Autodesk Inventor part; units mm, degrees
(part 2 of 2)
sketch "Sketch3" plane through (0, 0, -3.4) normal (0, 0, -1) x (-1, 0, 0)
  line L0 (0, 0.65) -> (23.75, 0.65)
  line L1 (23.75, 0.65) -> (23.75, 66.4871)
  line L2 (23.75, 66.4871) -> (0, 66.4871)
  line L3 (0, 66.4871) -> (0, 0.65)
  circle A0 centre (13, 35.9222) radius 9.6 construction
  circle A1 centre (9.652, 48.0693) radius 8 construction
  circle A2 centre (9.652, 48.0693) radius 8.4
  circle A3 centre (13, 35.9222) radius 10
  circle A4 centre (15.35, 56.2871) radius 5 projected
  circle A5 centre (9.652, 48.0693) radius 1.25 construction
  arc A6 (10.4245, 56.0319) -> (9.9568, 54.9375) centre (14.7581, 53.5328) ccw construction
  arc A7 (9.9568, 54.9375) -> (9.5969, 54.944) centre (9.652, 48.0693) ccw construction
  arc A8 (9.5969, 54.944) -> (9.1694, 56.0547) centre (4.7478, 53.7148) ccw construction
  arc A9 (9.1694, 56.0547) -> (8.7521, 56.0185) centre (9.652, 48.0693) ccw construction
  arc A10 (8.7521, 56.0185) -> (8.5222, 54.8508) centre (13.5106, 54.4751) ccw construction
  arc A11 (8.5222, 54.8508) -> (8.1688, 54.7824) centre (9.652, 48.0693) ccw construction
  arc A12 (8.1688, 54.7824) -> (7.5196, 55.7798) centre (3.6812, 52.5718) ccw construction
  arc A13 (7.5196, 55.7798) -> (7.119, 55.6577) centre (9.652, 48.0693) ccw construction
  arc A14 (7.119, 55.6577) -> (7.1369, 54.4677) centre (12.0944, 55.1373) ccw construction
  arc A15 (7.1369, 54.4677) -> (6.8055, 54.3273) centre (9.652, 48.0693) ccw construction
  arc A16 (6.8055, 54.3273) -> (5.9631, 55.168) centre (2.8755, 51.232) ccw construction
  arc A17 (5.9631, 55.168) -> (5.5966, 54.9652) centre (9.652, 48.0693) ccw construction
  arc A18 (5.5966, 54.9652) -> (5.8615, 53.805) centre (10.5715, 55.4907) ccw construction
  arc A19 (5.8615, 53.805) -> (5.5666, 53.5987) centre (9.652, 48.0693) ccw construction
  arc A20 (5.5666, 53.5987) -> (4.5678, 54.2459) centre (2.366, 49.754) ccw construction
  arc A21 (4.5678, 54.2459) -> (4.2515, 53.9714) centre (9.652, 48.0693) ccw construction
  arc A22 (4.2515, 53.9714) -> (4.7519, 52.8916) centre (9.0084, 55.5197) ccw construction
  arc A23 (4.7519, 52.8916) -> (4.5062, 52.6285) centre (9.652, 48.0693) ccw construction
  arc A24 (4.5062, 52.6285) -> (3.3947, 53.0539) centre (2.175, 48.2023) ccw construction
  arc A25 (3.3947, 53.0539) -> (3.1424, 52.7196) centre (9.652, 48.0693) ccw construction
  arc A26 (3.1424, 52.7196) -> (3.8563, 51.7674) centre (7.4735, 55.2231) ccw construction
  arc A27 (3.8563, 51.7674) -> (3.6707, 51.459) centre (9.652, 48.0693) ccw construction
  arc A28 (3.6707, 51.459) -> (2.4951, 51.644) centre (2.3107, 46.6449) ccw construction
  arc A29 (2.4951, 51.644) -> (2.3178, 51.2646) centre (9.652, 48.0693) ccw construction
  arc A30 (2.3178, 51.2646) -> (3.2141, 50.4816) centre (6.0337, 54.6138) ccw construction
  arc A31 (3.2141, 50.4816) -> (3.0967, 50.1413) centre (9.652, 48.0693) ccw construction
  arc A32 (3.0967, 50.1413) -> (1.9082, 50.0779) centre (2.7673, 45.1497) ccw construction
  arc A33 (1.9082, 50.0779) -> (1.8137, 49.6699) centre (9.652, 48.0693) ccw construction
  arc A34 (1.8137, 49.6699) -> (2.8532, 49.0904) centre (4.7521, 53.7185) ccw construction
  arc A35 (2.8532, 49.0904) -> (2.8091, 48.7331) centre (9.652, 48.0693) ccw construction
  arc A36 (2.8091, 48.7331) -> (1.6598, 48.424) centre (3.5247, 43.7821) ccw construction
  arc A37 (1.6598, 48.424) -> (1.6522, 48.0052) centre (9.652, 48.0693) ccw construction
  arc A38 (1.6522, 48.0052) -> (2.7895, 47.6545) centre (3.6846, 52.5763) ccw construction
  arc A39 (2.7895, 47.6545) -> (2.8206, 47.2959) centre (9.652, 48.0693) ccw construction
  arc A40 (2.8206, 47.2959) -> (1.7607, 46.7546) centre (4.55, 42.6018) ccw construction
  arc A41 (1.7607, 46.7546) -> (1.8404, 46.3434) centre (9.652, 48.0693) ccw construction
  arc A42 (1.8404, 46.3434) -> (3.0257, 46.2368) centre (2.8779, 51.2371) ccw construction
  arc A43 (3.0257, 46.2368) -> (3.1307, 45.8925) centre (9.652, 48.0693) ccw construction
  arc A44 (3.1307, 45.8925) -> (2.2065, 45.1426) centre (5.7982, 41.6605) ccw construction
  arc A45 (2.2065, 45.1426) -> (2.3699, 44.757) centre (9.652, 48.0693) ccw construction
  arc A46 (2.3699, 44.757) -> (3.5515, 44.8991) centre (2.3673, 49.7595) ccw construction
  arc A47 (3.5515, 44.8991) -> (3.7258, 44.5842) centre (9.652, 48.0693) ccw construction
  arc A48 (3.7258, 44.5842) -> (2.9777, 43.6586) centre (7.2149, 40.9993) ccw construction
  arc A49 (2.9777, 43.6586) -> (3.2177, 43.3153) centre (9.652, 48.0693) ccw construction
  arc A50 (3.2177, 43.3153) -> (4.3439, 43.7001) centre (2.1751, 48.208) ccw construction
  arc A51 (4.3439, 43.7001) -> (4.5798, 43.4282) centre (9.652, 48.0693) ccw construction
  arc A52 (4.5798, 43.4282) -> (4.0406, 42.3673) centre (8.7381, 40.6471) ccw construction
  arc A53 (4.0406, 42.3673) -> (4.3467, 42.0814) centre (9.652, 48.0693) ccw construction
  arc A54 (4.3467, 42.0814) -> (5.3683, 42.6919) centre (2.3096, 46.6504) ccw construction
  arc A55 (5.3683, 42.6919) -> (5.6556, 42.4751) centre (9.652, 48.0693) ccw construction
  arc A56 (5.6556, 42.4751) -> (5.3487, 41.3252) centre (10.3012, 40.6193) ccw construction
  arc A57 (5.3487, 41.3252) -> (5.7076, 41.1093) centre (9.652, 48.0693) ccw construction
  arc A58 (5.7076, 41.1093) -> (6.5799, 41.9188) centre (2.7651, 45.1549) ccw construction
  arc A59 (6.5799, 41.9188) -> (6.906, 41.7665) centre (9.652, 48.0693) ccw construction
  arc A60 (6.906, 41.7665) -> (6.8449, 40.5779) centre (11.8359, 40.9171) ccw construction
  arc A61 (6.8449, 40.5779) -> (7.2408, 40.4413) centre (9.652, 48.0693) ccw construction
  arc A62 (7.2408, 40.4413) -> (7.9258, 41.4145) centre (3.5215, 43.7867) ccw construction
  arc A63 (7.9258, 41.4145) -> (8.2764, 41.3333) centre (9.652, 48.0693) ccw construction
  arc A64 (8.2764, 41.3333) -> (8.4638, 40.158) centre (13.2752, 41.5275) ccw construction
  arc A65 (8.4638, 40.158) -> (8.8795, 40.1066) centre (9.652, 48.0693) ccw construction
  arc A66 (8.8795, 40.1066) -> (9.3471, 41.201) centre (4.5458, 42.6057) ccw construction
  arc A67 (9.3471, 41.201) -> (9.707, 41.1945) centre (9.652, 48.0693) ccw construction
  arc A68 (9.707, 41.1945) -> (10.1346, 40.0838) centre (14.5562, 42.4237) ccw construction
  arc A69 (10.1346, 40.0838) -> (10.5519, 40.12) centre (9.652, 48.0693) ccw construction
  arc A70 (10.5519, 40.12) -> (10.7818, 41.2877) centre (5.7934, 41.6635) ccw construction
  arc A71 (10.7818, 41.2877) -> (11.1351, 41.3561) centre (9.652, 48.0693) ccw construction
  arc A72 (11.1351, 41.3561) -> (11.7843, 40.3587) centre (15.6228, 43.5667) ccw construction
  arc A73 (11.7843, 40.3587) -> (12.1849, 40.4808) centre (9.652, 48.0693) ccw construction
  arc A74 (12.1849, 40.4808) -> (12.167, 41.6708) centre (7.2095, 41.0012) ccw construction
  arc A75 (12.167, 41.6708) -> (12.4985, 41.8112) centre (9.652, 48.0693) ccw construction
  arc A76 (12.4985, 41.8112) -> (13.3408, 40.9705) centre (16.4284, 44.9065) ccw construction
  arc A77 (13.3408, 40.9705) -> (13.7073, 41.1733) centre (9.652, 48.0693) ccw construction
  arc A78 (13.7073, 41.1733) -> (13.4424, 42.3336) centre (8.7324, 40.6478) ccw construction
  arc A79 (13.4424, 42.3336) -> (13.7374, 42.5398) centre (9.652, 48.0693) ccw construction
  arc A80 (13.7374, 42.5398) -> (14.7361, 41.8926) centre (16.9379, 46.3845) ccw construction
  arc A81 (14.7361, 41.8926) -> (15.0524, 42.1671) centre (9.652, 48.0693) ccw construction
  arc A82 (15.0524, 42.1671) -> (14.5521, 43.247) centre (10.2955, 40.6188) ccw construction
  arc A83 (14.5521, 43.247) -> (14.7977, 43.51) centre (9.652, 48.0693) ccw construction
  arc A84 (14.7977, 43.51) -> (15.9092, 43.0846) centre (17.129, 47.9362) ccw construction
  arc A85 (15.9092, 43.0846) -> (16.1615, 43.4189) centre (9.652, 48.0693) ccw construction
  arc A86 (16.1615, 43.4189) -> (15.4476, 44.3711) centre (11.8305, 40.9154) ccw construction
  arc A87 (15.4476, 44.3711) -> (15.6332, 44.6795) centre (9.652, 48.0693) ccw construction
  arc A88 (15.6332, 44.6795) -> (16.8089, 44.4945) centre (16.9932, 49.4936) ccw construction
  arc A89 (16.8089, 44.4945) -> (16.9861, 44.874) centre (9.652, 48.0693) ccw construction
  arc A90 (16.9861, 44.874) -> (16.0899, 45.6569) centre (13.2702, 41.5247) ccw construction
  arc A91 (16.0899, 45.6569) -> (16.2073, 45.9972) centre (9.652, 48.0693) ccw construction
  arc A92 (16.2073, 45.9972) -> (17.3957, 46.0606) centre (16.5367, 50.9889) ccw construction
  arc A93 (17.3957, 46.0606) -> (17.4902, 46.4687) centre (9.652, 48.0693) ccw construction
  arc A94 (17.4902, 46.4687) -> (16.4507, 47.0482) centre (14.5519, 42.42) ccw construction
  arc A95 (16.4507, 47.0482) -> (16.4948, 47.4054) centre (9.652, 48.0693) ccw construction
  arc A96 (16.4948, 47.4054) -> (17.6441, 47.7145) centre (15.7792, 52.3565) ccw construction
  arc A97 (17.6441, 47.7145) -> (17.6517, 48.1333) centre (9.652, 48.0693) ccw construction
  arc A98 (17.6517, 48.1333) -> (16.5144, 48.484) centre (15.6193, 43.5622) ccw construction
  arc A99 (16.5144, 48.484) -> (16.4833, 48.8426) centre (9.652, 48.0693) ccw construction
  arc A100 (16.4833, 48.8426) -> (17.5432, 49.3839) centre (14.7539, 53.5367) ccw construction
  arc A101 (17.5432, 49.3839) -> (17.4636, 49.7951) centre (9.652, 48.0693) ccw construction
  arc A102 (17.4636, 49.7951) -> (16.2783, 49.9017) centre (16.426, 44.9014) ccw construction
  arc A103 (16.2783, 49.9017) -> (16.1733, 50.246) centre (9.652, 48.0693) ccw construction
  arc A104 (16.1733, 50.246) -> (17.0974, 50.9959) centre (13.5057, 54.478) ccw construction
  arc A105 (17.0974, 50.9959) -> (16.9341, 51.3815) centre (9.652, 48.0693) ccw construction
  arc A106 (16.9341, 51.3815) -> (15.7525, 51.2394) centre (16.9366, 46.379) ccw construction
  arc A107 (15.7525, 51.2394) -> (15.5782, 51.5543) centre (9.652, 48.0693) ccw construction
  arc A108 (15.5782, 51.5543) -> (16.3262, 52.4799) centre (12.089, 55.1392) ccw construction
  arc A109 (16.3262, 52.4799) -> (16.0863, 52.8232) centre (9.652, 48.0693) ccw construction
  arc A110 (16.0863, 52.8232) -> (14.96, 52.4385) centre (17.1289, 47.9305) ccw construction
  arc A111 (14.96, 52.4385) -> (14.7241, 52.7103) centre (9.652, 48.0693) ccw construction
  arc A112 (14.7241, 52.7103) -> (15.2634, 53.7712) centre (10.5659, 55.4914) ccw construction
  arc A113 (15.2634, 53.7712) -> (14.9573, 54.0571) centre (9.652, 48.0693) ccw construction
  arc A114 (14.9573, 54.0571) -> (13.9356, 53.4466) centre (16.9943, 49.4881) ccw construction
  arc A115 (13.9356, 53.4466) -> (13.6483, 53.6634) centre (9.652, 48.0693) ccw construction
  arc A116 (13.6483, 53.6634) -> (13.9552, 54.8133) centre (9.0028, 55.5192) ccw construction
  arc A117 (13.9552, 54.8133) -> (13.5964, 55.0293) centre (9.652, 48.0693) ccw construction
  arc A118 (13.5964, 55.0293) -> (12.724, 54.2197) centre (16.5389, 50.9836) ccw construction
  arc A119 (12.724, 54.2197) -> (12.3979, 54.3721) centre (9.652, 48.0693) ccw construction
  arc A120 (12.3979, 54.3721) -> (12.459, 55.5606) centre (7.468, 55.2214) ccw construction
  arc A121 (12.459, 55.5606) -> (12.0631, 55.6973) centre (9.652, 48.0693) ccw construction
  arc A122 (12.0631, 55.6973) -> (11.3781, 54.724) centre (15.7825, 52.3518) ccw construction
  arc A123 (11.3781, 54.724) -> (11.0275, 54.8052) centre (9.652, 48.0693) ccw construction
  arc A124 (11.0275, 54.8052) -> (10.8402, 55.9805) centre (6.0287, 54.6111) ccw construction
  arc A125 (10.8402, 55.9805) -> (10.4245, 56.0319) centre (9.652, 48.0693) ccw construction
  arc A126 (10.4239, 28.0847) -> (10.4838, 26.6578) centre (16.409, 27.6212) ccw construction
  arc A127 (10.4838, 26.6578) -> (10.9721, 26.5388) centre (13, 35.9222) ccw construction
  arc A128 (10.9721, 26.5388) -> (11.6817, 27.7782) centre (6.1543, 30.12) ccw construction
  arc A129 (11.6817, 27.7782) -> (12.1097, 27.7204) centre (13, 35.9222) ccw construction
  arc A130 (12.1097, 27.7204) -> (12.465, 26.3371) centre (18.0604, 28.5113) ccw construction
  arc A131 (12.465, 26.3371) -> (12.9673, 26.3223) centre (13, 35.9222) ccw construction
  arc A132 (12.9673, 26.3223) -> (13.4037, 27.6821) centre (7.5102, 28.8235) ccw construction
  arc A133 (13.4037, 27.6821) -> (13.8344, 27.7145) centre (13, 35.9222) ccw construction
  arc A134 (13.8344, 27.7145) -> (14.4695, 26.4353) centre (19.4907, 29.7254) ccw construction
  arc A135 (14.4695, 26.4353) -> (14.964, 26.5253) centre (13, 35.9222) ccw construction
  arc A136 (14.964, 26.5253) -> (15.1081, 27.9461) centre (9.1061, 27.8373) ccw construction
  arc A137 (15.1081, 27.9461) -> (15.5227, 28.0674) centre (13, 35.9222) ccw construction
  arc A138 (15.5227, 28.0674) -> (16.4098, 26.9482) centre (20.6372, 31.2103) ccw construction
  arc A139 (16.4098, 26.9482) -> (16.8748, 27.1389) centre (13, 35.9222) ccw construction
  arc A140 (16.8748, 27.1389) -> (16.7204, 28.5587) centre (10.8721, 27.2043) ccw construction
  arc A141 (16.7204, 28.5587) -> (17.1007, 28.7635) centre (13, 35.9222) ccw construction
  arc A142 (17.1007, 28.7635) -> (18.2011, 27.8532) centre (21.45, 32.9011) ccw construction
  arc A143 (18.2011, 27.8532) -> (18.6163, 28.1365) centre (13, 35.9222) ccw construction
  arc A144 (18.6163, 28.1365) -> (18.17, 29.4931) centre (12.7312, 26.9524) ccw construction
  arc A145 (18.17, 29.4931) -> (18.4994, 29.7725) centre (13, 35.9222) ccw construction
  arc A146 (18.4994, 29.7725) -> (19.7651, 29.1109) centre (21.8934, 34.724) ccw construction
  arc A147 (19.7651, 29.1109) -> (20.1123, 29.4743) centre (13, 35.9222) ccw construction
  arc A148 (20.1123, 29.4743) -> (19.3937, 30.7085) centre (14.602, 27.0926) ccw construction
  arc A149 (19.3937, 30.7085) -> (19.6578, 31.0503) centre (13, 35.9222) ccw construction
  arc A150 (19.6578, 31.0503) -> (21.0334, 30.6663) centre (21.9482, 36.5992) ccw construction
  arc A151 (21.0334, 30.6663) -> (21.2975, 31.0939) centre (13, 35.9222) ccw construction
  arc A152 (21.2975, 31.0939) -> (20.338, 32.1518) centre (16.4027, 27.6186) ccw construction
  arc A153 (20.338, 32.1518) -> (20.5253, 32.541) centre (13, 35.9222) ccw construction
  arc A154 (20.5253, 32.541) -> (21.9506, 32.4514) centre (21.6119, 38.4449) ccw construction
  arc A155 (21.9506, 32.4514) -> (22.12, 32.9246) centre (13, 35.9222) ccw construction
  arc A156 (22.12, 32.9246) -> (20.9616, 33.7599) centre (18.0548, 28.5075) ccw construction
  arc A157 (20.9616, 33.7599) -> (21.0638, 34.1795) centre (13, 35.9222) ccw construction
  arc A158 (21.0638, 34.1795) -> (22.4766, 34.3882) centre (20.8992, 40.1803) ccw construction
  arc A159 (22.4766, 34.3882) -> (22.5439, 34.8863) centre (13, 35.9222) ccw construction
  arc A160 (22.5439, 34.8863) -> (21.2372, 35.4624) centre (19.486, 29.7205) ccw construction
  arc A161 (21.2372, 35.4624) -> (21.25, 35.8941) centre (13, 35.9222) ccw construction
  arc A162 (21.25, 35.8941) -> (22.5885, 36.392) centre (19.8413, 41.7296) ccw construction
  arc A163 (22.5885, 36.392) -> (22.5508, 36.8932) centre (13, 35.9222) ccw construction
  arc A164 (22.5508, 36.8932) -> (21.1528, 37.1851) centre (20.6336, 31.2045) ccw construction
  arc A165 (21.1528, 37.1851) -> (21.0755, 37.61) centre (13, 35.9222) ccw construction
  arc A166 (21.0755, 37.61) -> (22.2813, 38.3753) centre (18.4844, 43.0251) ccw construction
  arc A167 (22.2813, 38.3753) -> (22.1402, 38.8577) centre (13, 35.9222) ccw construction
  arc A168 (22.1402, 38.8577) -> (20.7121, 38.8525) centre (21.4477, 32.8947) ccw construction
  arc A169 (20.7121, 38.8525) -> (20.5481, 39.2521) centre (13, 35.9222) ccw construction
  arc A170 (20.5481, 39.2521) -> (21.5684, 40.2514) centre (16.8878, 44.0101) ccw construction
  arc A171 (21.5684, 40.2514) -> (21.3301, 40.6939) centre (13, 35.9222) ccw construction
  arc A172 (21.3301, 40.6939) -> (19.9343, 40.3919) centre (21.8925, 34.7172) ccw construction
  arc A173 (19.9343, 40.3919) -> (19.6909, 40.7487) centre (13, 35.9222) ccw construction
  arc A174 (19.6909, 40.7487) -> (20.4811, 41.9383) centre (15.1213, 44.6417) ccw construction
  arc A175 (20.4811, 41.9383) -> (20.156, 42.3216) centre (13, 35.9222) ccw construction
  arc A176 (20.156, 42.3216) -> (18.8534, 41.736) centre (21.9487, 36.5924) ccw construction
  arc A177 (18.8534, 41.736) -> (18.5412, 42.0343) centre (13, 35.9222) ccw construction
  arc A178 (18.5412, 42.0343) -> (19.0668, 43.3622) centre (13.262, 44.8922) ccw construction
  arc A179 (19.0668, 43.3622) -> (18.6691, 43.6695) centre (13, 35.9222) ccw construction
  arc A180 (18.6691, 43.6695) -> (17.5168, 42.8259) centre (21.6138, 38.4383) ccw construction
  arc A181 (17.5168, 42.8259) -> (17.1493, 43.0528) centre (13, 35.9222) ccw construction
  arc A182 (17.1493, 43.0528) -> (17.3874, 44.461) centre (11.3913, 44.7507) ccw construction
  arc A183 (17.3874, 44.461) -> (16.9345, 44.6789) centre (13, 35.9222) ccw construction
  arc A184 (16.9345, 44.6789) -> (15.9827, 43.6141) centre (20.9025, 40.1743) ccw construction
  arc A185 (15.9827, 43.6141) -> (15.5761, 43.7597) centre (13, 35.9222) ccw construction
  arc A186 (15.5761, 43.7597) -> (15.5162, 45.1866) centre (9.591, 44.2233) ccw construction
  arc A187 (15.5162, 45.1866) -> (15.0279, 45.3056) centre (13, 35.9222) ccw construction
  arc A188 (15.0279, 45.3056) -> (14.3183, 44.0662) centre (19.8457, 41.7244) ccw construction
  arc A189 (14.3183, 44.0662) -> (13.8903, 44.124) centre (13, 35.9222) ccw construction
  arc A190 (13.8903, 44.124) -> (13.535, 45.5073) centre (7.9396, 43.3331) ccw construction
  arc A191 (13.535, 45.5073) -> (13.0327, 45.5222) centre (13, 35.9222) ccw construction
  arc A192 (13.0327, 45.5222) -> (12.5963, 44.1623) centre (18.4898, 43.0209) ccw construction
  arc A193 (12.5963, 44.1623) -> (12.1656, 44.1299) centre (13, 35.9222) ccw construction
  arc A194 (12.1656, 44.1299) -> (11.5305, 45.4091) centre (6.5093, 42.119) ccw construction
  arc A195 (11.5305, 45.4091) -> (11.036, 45.3192) centre (13, 35.9222) ccw construction
  arc A196 (11.036, 45.3192) -> (10.8919, 43.8983) centre (16.8939, 44.0072) ccw construction
  arc A197 (10.8919, 43.8983) -> (10.4773, 43.7771) centre (13, 35.9222) ccw construction
  arc A198 (10.4773, 43.7771) -> (9.5902, 44.8962) centre (5.3628, 40.6341) ccw construction
  arc A199 (9.5902, 44.8962) -> (9.1252, 44.7055) centre (13, 35.9222) ccw construction
  arc A200 (9.1252, 44.7055) -> (9.2796, 43.2857) centre (15.1279, 44.6401) ccw construction
  arc A201 (9.2796, 43.2857) -> (8.8993, 43.0809) centre (13, 35.9222) ccw construction
  arc A202 (8.8993, 43.0809) -> (7.7989, 43.9912) centre (4.55, 38.9433) ccw construction
  arc A203 (7.7989, 43.9912) -> (7.3837, 43.7079) centre (13, 35.9222) ccw construction
  arc A204 (7.3837, 43.7079) -> (7.83, 42.3513) centre (13.2688, 44.892) ccw construction
  arc A205 (7.83, 42.3513) -> (7.5006, 42.0719) centre (13, 35.9222) ccw construction
  arc A206 (7.5006, 42.0719) -> (6.2349, 42.7335) centre (4.1066, 37.1204) ccw construction
  arc A207 (6.2349, 42.7335) -> (5.8877, 42.3701) centre (13, 35.9222) ccw construction
  arc A208 (5.8877, 42.3701) -> (6.6063, 41.1359) centre (11.398, 44.7519) ccw construction
  arc A209 (6.6063, 41.1359) -> (6.3422, 40.7941) centre (13, 35.9222) ccw construction
  arc A210 (6.3422, 40.7941) -> (4.9666, 41.1781) centre (4.0518, 35.2452) ccw construction
  arc A211 (4.9666, 41.1781) -> (4.7025, 40.7505) centre (13, 35.9222) ccw construction
  arc A212 (4.7025, 40.7505) -> (5.662, 39.6926) centre (9.5973, 44.2259) ccw construction
  arc A213 (5.662, 39.6926) -> (5.4747, 39.3034) centre (13, 35.9222) ccw construction
  arc A214 (5.4747, 39.3034) -> (4.0494, 39.393) centre (4.3881, 33.3995) ccw construction
  arc A215 (4.0494, 39.393) -> (3.88, 38.9198) centre (13, 35.9222) ccw construction
  arc A216 (3.88, 38.9198) -> (5.0384, 38.0846) centre (7.9452, 43.3369) ccw construction
  arc A217 (5.0384, 38.0846) -> (4.9362, 37.6649) centre (13, 35.9222) ccw construction
  arc A218 (4.9362, 37.6649) -> (3.5234, 37.4562) centre (5.1008, 31.6641) ccw construction
  arc A219 (3.5234, 37.4562) -> (3.4561, 36.9582) centre (13, 35.9222) ccw construction
  arc A220 (3.4561, 36.9582) -> (4.7628, 36.382) centre (6.514, 42.124) ccw construction
  arc A221 (4.7628, 36.382) -> (4.75, 35.9503) centre (13, 35.9222) ccw construction
  arc A222 (4.75, 35.9503) -> (3.4115, 35.4524) centre (6.1587, 30.1148) ccw construction
  arc A223 (3.4115, 35.4524) -> (3.4492, 34.9512) centre (13, 35.9222) ccw construction
  arc A224 (3.4492, 34.9512) -> (4.8472, 34.6594) centre (5.3664, 40.6399) ccw construction
  arc A225 (4.8472, 34.6594) -> (4.9245, 34.2344) centre (13, 35.9222) ccw construction
  arc A226 (4.9245, 34.2344) -> (3.7187, 33.4691) centre (7.5156, 28.8194) ccw construction
  arc A227 (3.7187, 33.4691) -> (3.8598, 32.9867) centre (13, 35.9222) ccw construction
  arc A228 (3.8598, 32.9867) -> (5.2879, 32.9919) centre (4.5523, 38.9497) ccw construction
  arc A229 (5.2879, 32.9919) -> (5.4519, 32.5923) centre (13, 35.9222) ccw construction
  arc A230 (5.4519, 32.5923) -> (4.4316, 31.593) centre (9.1122, 27.8343) ccw construction
  arc A231 (4.4316, 31.593) -> (4.6699, 31.1505) centre (13, 35.9222) ccw construction
  arc A232 (4.6699, 31.1505) -> (6.0657, 31.4525) centre (4.1075, 37.1272) ccw construction
  arc A233 (6.0657, 31.4525) -> (6.3091, 31.0957) centre (13, 35.9222) ccw construction
  arc A234 (6.3091, 31.0957) -> (5.5189, 29.9062) centre (10.8787, 27.2027) ccw construction
  arc A235 (5.5189, 29.9062) -> (5.844, 29.5229) centre (13, 35.9222) ccw construction
  arc A236 (5.844, 29.5229) -> (7.1466, 30.1085) centre (4.0513, 35.252) ccw construction
  arc A237 (7.1466, 30.1085) -> (7.4588, 29.8101) centre (13, 35.9222) ccw construction
  arc A238 (7.4588, 29.8101) -> (6.9332, 28.4822) centre (12.738, 26.9522) ccw construction
  arc A239 (6.9332, 28.4822) -> (7.3309, 28.1749) centre (13, 35.9222) ccw construction
  arc A240 (7.3309, 28.1749) -> (8.4832, 29.0185) centre (4.3862, 33.4061) ccw construction
  arc A241 (8.4832, 29.0185) -> (8.8507, 28.7916) centre (13, 35.9222) ccw construction
  arc A242 (8.8507, 28.7916) -> (8.6126, 27.3834) centre (14.6087, 27.0938) ccw construction
  arc A243 (8.6126, 27.3834) -> (9.0655, 27.1655) centre (13, 35.9222) ccw construction
  arc A244 (9.0655, 27.1655) -> (10.0173, 28.2303) centre (5.0975, 31.6701) ccw construction
  arc A245 (10.0173, 28.2303) -> (10.4239, 28.0847) centre (13, 35.9222) ccw construction
  circle A246 centre (15.35, 15.35) radius 14.7 projected
  point P0 (16.9228, 44.7322)
  point P1 (4.6044, 41.3549)
  point P2 (17.4267, 44.8891)
  point P3 (17.5061, 49.5901)
  point P4 (17.2457, 51.6604)
  point P5 (10.3523, 56.44)
  dimension "d21" = 0.4
  dimension "d22" = 0.4
  dimension "d146" = 0
  constraints: 8 end point, 3 centre point, 3 point on circle, 2 coincident, 2 parallel, 1 horizontal, 1 perpendicular, 3 other
  measures "d21" radial gap between concentric circles of A1 A2
  measures "d146" distance edge to line of A246 L0
extrude "Extrusion7" add sketch "Sketch3" along normal blind 3.7 contours L3 L2 L1 A246 A3 A2 A4 L0 | A246 L1 L0 | A246 A3 L1
sketch "Sketch12" plane through (-34.0123, 35.7835, 2.1) normal (0, 0, -1) x (-0.6427876, 0.7660444, 0)
  circle A0 centre (-6.2471, 26.5582) radius 1.25 construction
  arc A1 (-8.6736, 23.1301) -> (-7.5759, 24.037) centre (-10.4403, 26.3862) ccw construction
  arc A2 (-7.5759, 24.037) -> (-7.2355, 23.8851) centre (-6.2471, 26.5582) ccw construction
  arc A3 (-7.2355, 23.8851) -> (-7.177, 22.4625) centre (-3.5738, 23.3231) ccw construction
  arc A4 (-7.177, 22.4625) -> (-6.6344, 22.3761) centre (-6.2471, 26.5582) ccw construction
  arc A5 (-6.6344, 22.3761) -> (-6.1373, 23.7104) centre (-9.7925, 24.3127) ccw construction
  arc A6 (-6.1373, 23.7104) -> (-5.7665, 23.7491) centre (-6.2471, 26.5582) ccw construction
  arc A7 (-5.7665, 23.7491) -> (-5.0045, 22.5463) centre (-2.3144, 25.0932) ccw construction
  arc A8 (-5.0045, 22.5463) -> (-4.4915, 22.7428) centre (-6.2471, 26.5582) ccw construction
  arc A9 (-4.4915, 22.7428) -> (-4.728, 24.1468) centre (-8.1948, 22.8408) ccw construction
  arc A10 (-4.728, 24.1468) -> (-4.4263, 24.3657) centre (-6.2471, 26.5582) ccw construction
  arc A11 (-4.4263, 24.3657) -> (-3.165, 23.705) centre (-2.1087, 27.2558) ccw construction
  arc A12 (-3.165, 23.705) -> (-2.819, 24.1317) centre (-6.2471, 26.5582) ccw construction
  arc A13 (-2.819, 24.1317) -> (-3.7259, 25.2294) centre (-6.0751, 22.365) ccw construction
  arc A14 (-3.7259, 25.2294) -> (-3.574, 25.5699) centre (-6.2471, 26.5582) ccw construction
  arc A15 (-3.574, 25.5699) -> (-2.1513, 25.6283) centre (-3.012, 29.2315) ccw construction
  arc A16 (-2.1513, 25.6283) -> (-2.065, 26.1709) centre (-6.2471, 26.5582) ccw construction
  arc A17 (-2.065, 26.1709) -> (-3.3992, 26.6681) centre (-4.0015, 23.0128) ccw construction
  arc A18 (-3.3992, 26.6681) -> (-3.4379, 27.0389) centre (-6.2471, 26.5582) ccw construction
  arc A19 (-3.4379, 27.0389) -> (-2.2351, 27.8008) centre (-4.782, 30.491) ccw construction
  arc A20 (-2.2351, 27.8008) -> (-2.4316, 28.3138) centre (-6.2471, 26.5582) ccw construction
  arc A21 (-2.4316, 28.3138) -> (-3.8357, 28.0773) centre (-2.5297, 24.6106) ccw construction
  arc A22 (-3.8357, 28.0773) -> (-4.0546, 28.3791) centre (-6.2471, 26.5582) ccw construction
  arc A23 (-4.0546, 28.3791) -> (-3.3939, 29.6403) centre (-6.9447, 30.6966) ccw construction
  arc A24 (-3.3939, 29.6403) -> (-3.8206, 29.9864) centre (-6.2471, 26.5582) ccw construction
  arc A25 (-3.8206, 29.9864) -> (-4.9183, 29.0795) centre (-2.0539, 26.7303) ccw construction
  arc A26 (-4.9183, 29.0795) -> (-5.2587, 29.2314) centre (-6.2471, 26.5582) ccw construction
  arc A27 (-5.2587, 29.2314) -> (-5.3172, 30.654) centre (-8.9204, 29.7934) ccw construction
  arc A28 (-5.3172, 30.654) -> (-5.8598, 30.7403) centre (-6.2471, 26.5582) ccw construction
  arc A29 (-5.8598, 30.7403) -> (-6.3569, 29.4061) centre (-2.7017, 28.8038) ccw construction
  arc A30 (-6.3569, 29.4061) -> (-6.7277, 29.3674) centre (-6.2471, 26.5582) ccw construction
  arc A31 (-6.7277, 29.3674) -> (-7.4897, 30.5702) centre (-10.1798, 28.0233) ccw construction
  arc A32 (-7.4897, 30.5702) -> (-8.0027, 30.3737) centre (-6.2471, 26.5582) ccw construction
  arc A33 (-8.0027, 30.3737) -> (-7.7662, 28.9697) centre (-4.2995, 30.2757) ccw construction
  arc A34 (-7.7662, 28.9697) -> (-8.0679, 28.7508) centre (-6.2471, 26.5582) ccw construction
  arc A35 (-8.0679, 28.7508) -> (-9.3292, 29.4114) centre (-10.3855, 25.8607) ccw construction
  arc A36 (-9.3292, 29.4114) -> (-9.6753, 28.9847) centre (-6.2471, 26.5582) ccw construction
  arc A37 (-9.6753, 28.9847) -> (-8.7684, 27.8871) centre (-6.4191, 30.7515) ccw construction
  arc A38 (-8.7684, 27.8871) -> (-8.9202, 27.5466) centre (-6.2471, 26.5582) ccw construction
  arc A39 (-8.9202, 27.5466) -> (-10.3429, 27.4881) centre (-9.4822, 23.8849) ccw construction
  arc A40 (-10.3429, 27.4881) -> (-10.4292, 26.9456) centre (-6.2471, 26.5582) ccw construction
  arc A41 (-10.4292, 26.9456) -> (-9.095, 26.4484) centre (-8.4927, 30.1037) ccw construction
  arc A42 (-9.095, 26.4484) -> (-9.0563, 26.0776) centre (-6.2471, 26.5582) ccw construction
  arc A43 (-9.0563, 26.0776) -> (-10.2591, 25.3157) centre (-7.7122, 22.6255) ccw construction
  arc A44 (-10.2591, 25.3157) -> (-10.0626, 24.8026) centre (-6.2471, 26.5582) ccw construction
  arc A45 (-10.0626, 24.8026) -> (-8.6585, 25.0392) centre (-9.9646, 28.5059) ccw construction
  arc A46 (-8.6585, 25.0392) -> (-8.4396, 24.7374) centre (-6.2471, 26.5582) ccw construction
  arc A47 (-8.4396, 24.7374) -> (-9.1003, 23.4761) centre (-5.5495, 22.4199) ccw construction
  arc A48 (-9.1003, 23.4761) -> (-8.6736, 23.1301) centre (-6.2471, 26.5582) ccw construction
  circle A49 centre (-6.2471, 26.5582) radius 4.2 construction
  circle A50 centre (-6.2471, 26.5582) radius 4.6
  point P0 (-49.2745, 3.0538)
  dimension "d128" = 0.4
  constraints: 1 centre point, 1 coincident, 3 other
extrude "Extrusion11" add sketch "Sketch12" along normal blind 1.5
ref_plane "Work Plane8" through (-34.0123, -5.0123, 0) normal (0, 0, -1) x (0.6427876, 0.7660444, 0)
sketch "Sketch4" plane through (0, 0, -7.1) normal (0, 0, -1) x (-1, 0, 0)
  line L0 (1.5, 1.65) -> (1.5, 17.65) projected
  line L1 (2.5, 1.65) -> (1.5, 1.65) projected
  line L2 (2.5, 17.65) -> (2.5, 1.65) projected
  line L3 (2.5, 17.65) -> (1.5, 17.65) projected
  line L4 (2.5, 17.65) -> (2.5, 18.15)
  line L5 (2.5, 18.15) -> (1, 18.15)
  line L6 (1, 18.15) -> (1, 1.65)
  line L7 (23.75, 0.65) -> (0, 0.65) projected
  line L8 (1, 1.65) -> (1.5, 1.65)
  point P0 (0, 0)
  dimension "d27" = 0.5
  dimension "d28" = 0.5
  constraints: 8 end point, 2 perpendicular, 1 collinear, 1 vertical
  measures "d27" distance between parallel lines of L5 L3
  measures "d28" distance between parallel lines of L6 L0
extrude "Extrusion8" cut sketch "Sketch4" against normal blind 7.1
sketch "Sketch9" plane through (-0.6572, 1.1216, 0.6) normal (0, 0, -1) x (-1, 0, 0)
  arc A0 (9.6951, 55.3184) -> (3.9472, 40.2333) centre (8.9947, 46.9477) ccw projected
  point P0 (-0.6572, -1.1216)
  point P1 (16.7695, 43.7675)
  point P2 (9.5001, 55.3324)
hole "Hole3" at (-9.652, 48.0693, 0.6) direction (0, 0, 1) diameter 2.5 depth 1.3
sketch "Sketch5" plane through (0, 0, -7.1) normal (0, 0, -1) x (-1, 0, 0)
  line L0 (1.5, 1.65) -> (1.5, 17.65) projected
  line L1 (2.5, 1.65) -> (1.5, 1.65) projected
  line L2 (2.5, 17.65) -> (2.5, 1.65) projected
  line L3 (2.5, 17.65) -> (1.5, 17.65) projected
  line L4 (2.5, 17.65) -> (2.5, 19.15)
  line L5 (2.5, 19.15) -> (0, 19.15)
  line L6 (0, 0) -> (0, 66.4871) projected
  line L7 (0, 0) -> (0, 19.15)
  line L8 (0, 0) -> (2.5, 0)
  line L9 (2.5, 0) -> (2.5, 1.65)
  line L10 (1, 18.15) -> (1, 1.15)
  line L11 (1, 1.15) -> (3, 1.15)
  line L12 (3, 1.15) -> (3, 18.15)
  line L13 (3, 18.15) -> (1, 18.15)
  line L14 (1.5, 14.55) -> (1.5, 11.05) projected
  line L15 (1.5, 14.55) -> (0, 14.55) projected
  line L16 (0, 11.05) -> (0, 14.55) projected
  line L17 (1.5, 11.05) -> (0, 11.05) projected
  line L18 (1.5, 8.25) -> (1.5, 4.75) projected
  line L19 (1.5, 8.25) -> (0, 8.25) projected
  line L20 (0, 4.75) -> (0, 8.25) projected
  line L21 (1.5, 4.75) -> (0, 4.75) projected
  line L22 (-0.5, 15.05) -> (2, 15.05)
  line L23 (2, 15.05) -> (2, 10.55)
  line L24 (2, 10.55) -> (-0.5, 10.55)
  line L25 (-0.5, 10.55) -> (-0.5, 15.05)
  line L26 (-0.5, 8.75) -> (2, 8.75)
  line L27 (2, 8.75) -> (2, 4.25)
  line L28 (2, 4.25) -> (-0.5, 4.25)
  line L29 (-0.5, 4.25) -> (-0.5, 8.75)
  line L30 (1.5, 1.65) -> (1, 1.65)
  point P0 (0, 15.05)
  point P1 (1, 15.05)
  point P2 (2.5, 18.15)
  point P3 (0, 8.75)
  point P4 (1, 8.75)
  point P5 (1, 10.55)
  point P6 (0, 10.55)
  point P7 (1, 4.25)
  point P8 (0, 4.25)
  point P9 (0, 4.25)
  point P10 (0, 8.75)
  point P11 (2.5, 1.15)
  point P12 (1, 0)
  dimension "d31" = 0.5
  dimension "d32" = 1
  dimension "d33" = 0.5
  dimension "d34" = 0.5
  constraints: 36 end point, 3 perpendicular, 3 point on line, 2 collinear, 1 vertical, 9 other
  measures "d31" distance between parallel lines of L0 L10
  measures "d32" distance between parallel lines of L5 L13
  measures "d33" distance between parallel lines of L15 L22
  measures "d34" distance between parallel lines of L19 L26
ref_plane "Work Plane6" through (-2.5, 0.5, -17) normal (0, 0, -1) x (0, 1, 0)
ref_plane "Work Plane9" through (-27.65, 0, -16.5) normal (0, 0, 1) x (1, 0, 0)
extrude "Extrusion9" add sketch "Sketch5" along normal up to surface (9.4 mm away) contours L1 L9 L11 L10 L30 | L10 L11 L9 L8 L6 L28 | L13 L10 L22 L6 L5 L4
sketch "Sketch7" plane through (0, 0, -7.1) normal (0, 0, -1) x (-1, 0, 0)
  circle A0 centre (9.6931, 61.9439) radius 1.0564 projected
  circle A1 centre (21.0069, 50.6302) radius 1.0564 projected
  circle A2 centre (15.35, 56.2871) radius 5 projected
  circle A3 centre (15.35, 56.2871) radius 14 projected
  circle A4 centre (9.6931, 61.9439) radius 2.25
  circle A5 centre (21.0069, 50.6302) radius 2.25
  point P0 (0, 0)
  dimension "d132" = 4.5
  dimension "d133" = 4.5
  constraints: 2 centre point, 2 coincident
  measures "d132" diameter of A4
  measures "d133" diameter of A5
extrude "Extrusion10" cut sketch "Sketch7" against normal blind 2.6 contours A0 | A1 | A4 | A5
sketch "Sketch8" plane through (-8.7501, 63.6888, -4.5) normal (0, 0, -1) x (-1, 0, 0)
  circle A0 centre (0.943, -1.7448) radius 1.0564 projected
  circle A1 centre (12.2567, -13.0586) radius 1.0564 projected
  circle A2 centre (6.5999, -7.4017) radius 5 projected
  circle A3 centre (6.5999, -7.4017) radius 14 projected
  point P0 (-8.7501, -63.6888)
  point P1 (0, 0)
  point P2 (12.2567, -10.2846)
hole "Hole2" at (-21.0069, 50.6302, -4.5) at (-9.6931, 61.9439, -4.5) direction (0, 0, 1) diameter 2.5 depth 8.8 counterbore diameter 4.5 counterbore depth 2.5
sketch "Sketch6" plane through (-23.75, 66.4871, 2.1) normal (0, 1, 0) x (1, 0, 0)
  line L0 (0, 9.2) -> (0, 0) projected
  line L1 (23.75, 0) -> (0, 0) projected
  line L2 (0, 4.6) -> (23.75, 4.6)
  line L3 (0.75, 9.2) -> (20.75, 9.2) projected
  line L4 (17.75, 9.2) -> (17.75, 0)
  circle A0 centre (11.25, 4.6) radius 3.5
  circle A1 centre (3.5, 4.6) radius 3.5
  line L5 (23.75, 9.2) -> (23.75, 0) projected
  line L6 (0, 9.2) -> (23.75, 9.2) projected
  point P0 (23.75, 2.1)
  point P1 (11.875, 4.6)
  point P2 (19.8, 4.6)
  point P3 (19.1456, 9.2)
  point P4 (6.3233, 9.2)
  dimension "d52" = 7
  dimension "d53" = 7
  dimension "d55" = 0
  dimension "d67" = 3
  dimension "d102" = 6
  constraints: 5 point on line, 4 end point, 3 midpoint, 2 centre point, 1 perpendicular
  measures "d52" diameter of A1
  measures "d53" diameter of A0
  measures "d55" distance edge to line of A1 L0
  measures "d67" distance edge to line of A0 L4
  measures "d102" distance between parallel lines of L5 L4
hole "Hole1" at (-20.25, 66.4871, -2.5) at (-12.5, 66.4871, -2.5) direction (0, -1, 0) diameter 4 depth 4 counterbore diameter 4.5 counterbore depth 0.5
sketch "Sketch10" plane through (0, 0, -7.1) normal (0, 0, -1) x (-1, 0, 0)
  line L0 (23.75, 0.65) -> (23.75, 66.4871) projected
  line L1 (23.75, 4.75) -> (0, 4.75)
  line L2 (0, 0) -> (0, 66.4871) projected
  line L3 (0, 13) -> (23.75, 13)
  line L4 (23.75, 19) -> (0, 19)
  circle A0 centre (3.5, 62.9871) radius 3.5
  circle A1 centre (3.5, 62.9871) radius 2.5
  line L5 (23.75, 66.4871) -> (0, 66.4871) projected
  line L6 (0, 66.4871) -> (0, 0) projected
  circle A2 centre (21.258, 45.6365) radius 3.5
  circle A3 centre (21.258, 45.6365) radius 2.75
  circle A4 centre (3.5, 26.3305) radius 3.5
  circle A5 centre (20.25, 22.5) radius 3.5
  line L7 (23.75, 0.65) -> (23.75, 66.4871) projected
  circle A6 centre (7, 8.875) radius 3.5
  circle A7 centre (19.75, 8.875) radius 3.5
  line L8 (23.75, 66.4871) -> (0, 66.4871) projected
  line L9 (0, 19.15) -> (2.5, 19.15) projected
  line L10 (1, 15.05) -> (0, 15.05) projected
  line L11 (0, 15.05) -> (0, 4.25) projected
  line L12 (0, 66.4871) -> (0, 19.15) projected
  circle A8 centre (9.6931, 61.9439) radius 2.25 projected
  circle A9 centre (21.0069, 50.6302) radius 2.25 projected
  line L13 (23.75, 0.65) -> (23.75, 66.4871) projected
  line L14 (23.75, 66.4871) -> (0, 66.4871) projected
  line L15 (0, 66.4871) -> (0, 19.15) projected
  line L16 (0, 19.15) -> (2.5, 19.15) projected
  arc A10 (17.2457, 51.6604) -> (10.3523, 56.44) centre (15.35, 56.2871) ccw projected
  arc A11 (17.4267, 44.8891) -> (17.2457, 51.6604) centre (9.652, 48.0693) ccw projected
  arc A12 (4.6044, 41.3549) -> (17.4267, 44.8891) centre (13, 35.9222) ccw projected
  arc A13 (10.3523, 56.44) -> (4.6044, 41.3549) centre (9.652, 48.0693) ccw projected
  arc A14 (4.6044, 41.3549) -> (17.4267, 44.8891) centre (13, 35.9222) ccw projected
  line L17 (2.5, 18.15) -> (2.5, 1.65) projected
  line L18 (2.5, 18.15) -> (2.5, 1.65) projected
  line L19 (0, 4.25) -> (1, 4.25) projected
  circle A15 centre (21.0069, 50.6302) radius 2.25 projected
  line L20 (2.5, 19.15) -> (2.5, 18.15) projected
  line L21 (2.5, 1.65) -> (2.5, 0.65) projected
  line L22 (1, 4.25) -> (1, 15.05) projected
  line L23 (2.5, 0.65) -> (23.75, 0.65) projected
  line L24 (2.5, 19.15) -> (2.5, 18.15) projected
  line L25 (2.5, 1.65) -> (2.5, 0.65) projected
  line L26 (1, 4.25) -> (1, 15.05) projected
  line L27 (2.5, 0.65) -> (23.75, 0.65) projected
  line L28 (1, 15.05) -> (0, 15.05) projected
  line L29 (0, 15.05) -> (0, 4.25) projected
  line L30 (0, 4.25) -> (1, 4.25) projected
  point P0 (23.2, 52.8075)
  point P1 (23.2, 54.1548)
  point P2 (23.2, -23.4755)
  point P3 (23.2, -18.5366)
  dimension "d77" = 8.25
  dimension "d78" = 6
  dimension "d79" = 7
  dimension "d80" = 5
  dimension "d81" = 7
  dimension "d82" = 5.5
  dimension "d86" = 7
  dimension "d87" = 7
  dimension "d88" = 7
  dimension "d89" = 7
  dimension "d90" = 4.125
  dimension "d91" = 4.125
  dimension "d92" = 7
  dimension "d93" = 4
  dimension "d94" = 4.125
  constraints: 8 centre point, 7 tangent, 6 end point, 6 point on line, 2 coincident, 1 horizontal, 1 perpendicular, 2 other
  measures "d77" distance between parallel lines of L3 L1
  measures "d78" distance between parallel lines of L3 L4
  measures "d79" diameter of A0
  measures "d80" diameter of A1
  measures "d81" diameter of A2
  measures "d82" diameter of A3
  measures "d86" diameter of A4
  measures "d87" diameter of A5
  measures "d88" diameter of A6
  measures "d89" distance from line of L2 A6.centre
  measures "d90" distance from line of L3 A6.centre
  measures "d91" distance from line of L1 A6.centre
  measures "d92" diameter of A7
  measures "d94" distance from line of L3 A7.centre
hole "Hole4" at (-3.5, 62.9871, -7.1) at (-21.258, 45.6365, -7.1) at (-20.25, 22.5, -7.1) at (-3.5, 26.3305, -7.1) at (-7, 8.875, -7.1) at (-19.75, 8.875, -7.1) direction (0, 0, 1) diameter 4 depth 3.5 counterbore diameter 4.5 counterbore depth 0.5
sketch "Sketch11" plane through (-23.75, 26.55, 2.1) normal (-1, 0, 0) x (0, 0, 1)
  circle A0 centre (-6.8505, -23.5505) radius 2.3495
  line L0 (-9.2, -25.9) -> (-9.2, 39.9371) projected
  line L1 (-2.1, -25.9) -> (0, -25.9) projected
  line L2 (-2.1, -6.2) -> (-2.1, -16.2) projected
  line L3 (-2.1, -17.2104) -> (-3.1, -17.2104) projected
  line L4 (-2.1, -6.3355) -> (-2.1, -22.4) projected
  line L5 (-2.1, -13.0104) -> (-9.2, -13.0104)
  line L6 (-9, 27.1271) -> (0, 27.1271)
  line L7 (0, 39.9371) -> (0, -25.9) projected
  circle A1 centre (-3, 32.901) radius 3
  line L8 (-8.7, 21.0865) -> (-8.7, 17.0865) projected
  line L9 (-5.7, 21.0865) -> (-5.7, 17.0865) projected
  line L10 (-9.2, 20.9848) -> (0, 20.9848)
  circle A2 centre (-3, 19.9848) radius 3
  line L11 (-8.7, -2.05) -> (-8.7, -6.05) projected
  line L12 (-5.7, -2.05) -> (-5.7, -6.05) projected
  line L13 (-9.2, 39.9371) -> (-9.2, -25.9) projected
  line L14 (-9.2, -0.7765) -> (-2.1, -0.7765)
  line L15 (-2.1, -6.3355) -> (-2.1, -22.4) projected
  line L16 (-5.5, -21.628) -> (-5.5, -17.2104) projected
  point P0 (-2.1, -26.55)
  point P1 (-6.1, -15.7765)
  point P2 (-6.1, -5.7765)
  point P3 (-5.65, -13.0104)
  point P4 (-3.9, 22.6271)
  point P5 (-9, 22.6271)
  point P6 (0, 0)
  point P7 (-8.7, 24.9848)
  point P8 (-8.7, 20.9848)
  point P9 (-5.2, 24.9848)
  point P10 (-5.2, 20.9848)
  point P11 (-8.5, -0.7765)
  point P12 (-8.5, -4.7765)
  point P13 (-6.6, -0.7765)
  point P14 (-6.6, -4.7765)
  point P15 (-9.2, -7.4)
  point P16 (-2.1, 0)
  point P17 (-2.1, -1.9431)
  point P18 (-5.2, 1.9975)
  point P19 (-5.2, -2.0025)
  point P20 (-6.1, 40.0194)
  point P21 (-5.5, -26.55)
  point P22 (-2.6, -1.801)
  point P23 (-2.6, -6.7398)
  point P24 (-5.2, 24.9848)
  point P25 (-8.7, 21.9971)
  point P26 (-8.7, 17.9971)
  point P27 (-5.2, 20.9848)
  point P28 (-5.7, 21.9971)
  point P29 (-5.7, 17.9971)
  dimension "d103" = 4.6989
  dimension "d104" = 4.2
  dimension "d105" = 3.55
  dimension "d106" = 3.55
  dimension "d107" = 6
  dimension "d109" = -6.2
  dimension "d110" = 6
  dimension "d113" = 1
  constraints: 8 end point, 6 point on line, 3 horizontal, 2 centre point, 2 tangent, 1 midpoint, 1 perpendicular, 10 other
  measures "d104" distance between parallel lines of L5 L3
  measures "d106" distance from line of L2 point (-5.65, -13.01)
  measures "d107" diameter of A1
  measures "d110" diameter of A2
  measures "d113" distance from line of A2.centre L10
hole "Hole5" at (-23.75, 13.5396, -3.55) at (-23.75, 46.5348, -0.9) at (-23.75, 59.451, -0.9) at (-23.75, 2.9995, -4.7505) direction (1, 0, 0) diameter 4 depth 3.5 counterbore diameter 4.5 counterbore depth 0.5
sketch "Sketch13" plane through (0, 0.65, 2.1) normal (1, 0, 0) x (0, 0, -1)
  line L0 (0, 28.1016) -> (0, 40.7924) projected
  line L1 (0, 40.7924) -> (-4.2, 40.7924) projected
  line L2 (-4.2, 28.1016) -> (-4.2, 40.7924) projected
  line L3 (0, 28.1016) -> (-4.2, 28.1016) projected
  ellipse E0 centre (-2.1, 37.6197) end of major axis (-0.1, 37.6197) minor radius 1.9381 projected
  ellipse E1 centre (-2.1, 31.2743) end of major axis (-0.1, 31.2743) minor radius 1.9381 projected
  point P0 (2.1, -0.65)
  point P1 (0, 47.7348)
  point P2 (0, 29.5207)
  point P3 (0, 34.3051)
  point P4 (0, 36.0687)
  point P5 (0, 40.853)
hole "Hole6" at (0, 38.2697, 4.2) at (0, 31.9243, 4.2) direction (-1, 0, 0) diameter 3.4 depth 8.8 countersink diameter 7 countersink angle 90 clearance for "Countersunk Flat Head Screw ISO 2009/7046" size "M3" standard "ISO"
chamfer "Chamfer1" distance 0.5 angle 45 2 edges at (-1, 15.05, -11.8) (-1, 4.25, -11.8)
body "Solid3"
